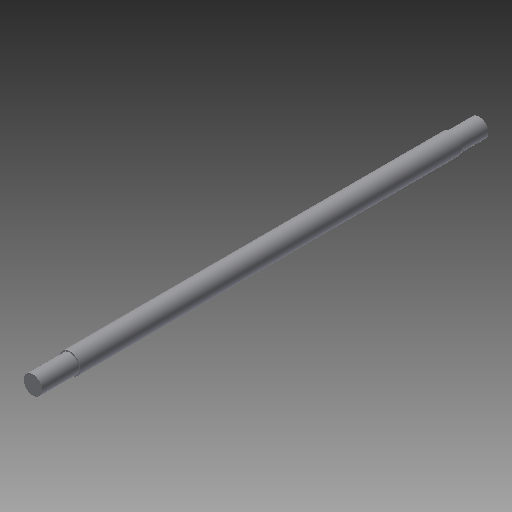
# Autodesk Inventor part: Welle
Saved by Autodesk Inventor 2018 (Build 220112000, 112)
## iProperties
Created: 2013-02-20
Part Number: Welle
Material: Generic
Document SubType Name: Modeling
Designer: Neef
Density: 1 g/cm^3
Appearance: Default
Author: Neef
Autodesk Inventor part; units mm, degrees
ref_plane "YZ Plane" through (0, 0, 0) normal (1, 0, 0) x (0, 1, 0)
ref_plane "XZ Plane" through (0, 0, 0) normal (0, 1, 0) x (-1, 0, 0)
ref_plane "XY Plane" through (0, 0, 0) normal (0, 0, 1) x (1, 0, 0)
sketch "Skizze1" plane through (0, 0, 0) normal (0, 0, 1) x (1, 0, 0)
  line L0 (0, 19.2) -> (0, -115.2) projected
  line L1 (-0.45, 0) -> (2.7, 0) projected
  line L2 (0, 0) -> (2, 0)
  line L3 (2.25, -6) -> (2.25, -88)
  line L4 (2.25, -88) -> (2, -88)
  line L5 (2, -88) -> (2, -96)
  line L6 (2, -96) -> (0, -96)
  line L7 (0, -96) -> (0, 0)
  line L8 (2, 0) -> (2, -6)
  line L9 (2, -6) -> (2.25, -6)
  point P0 (2.25, 0)
  dimension "d0" = 2
  dimension "d1" = 2.25
  dimension "d2" = 8
  dimension "d3" = 88
  dimension "d5" = 2
  dimension "d6" = 6
  constraints: 16 end point, 5 perpendicular, 2 point on line, 1 collinear, 1 parallel
  measures "d0" distance between parallel lines of L7 L5
  measures "d1" distance between parallel lines of L7 L3
  measures "d2" distance of L4.end L5.end
  measures "d3" distance of point (2.25, 0) L3.end
  measures "d5" distance between parallel lines of L0 L8
  measures "d6" distance of L2.end L8.end
revolve "Umdrehung1" add sketch "Skizze1" angle 360 about axis through (0, -96, 0) along (0, 1, 0)
